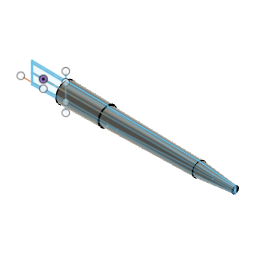
CustomDesignedTip_1000uL (Autodesk Fusion 360 design; units mm, degrees)
Autodesk Fusion 360 part; units mm, degrees
sketch "Sketch1" plane through (0, 0, 0) normal (0, 1, 0) x (1, 0, 0)
  line L0 (85.3, -0.9) -> (85.3, 0.9)
  line L1 (85.3, -1.4) -> (85.3, 1.4)
  line L2 (0, 0) -> (28.5, 0) construction
  line L3 (85.3, 0) -> (69.3, 0) construction
  line L4 (28.5, -4.086) -> (28.5, 4.086) construction
  line L5 (0, 0) -> (10, 0) construction
  line L6 (0, 3.75) -> (-10.0015, 3.75) construction
  line L7 (10, -3) -> (10, 3) construction
  line L8 (69.3, -3) -> (69.3, 3) construction
  line L9 (85.3, -0.9) -> (75.3, -0.9)
  line L10 (10, 3) -> (33, 3)
  line L11 (10, -3) -> (33, -3)
  line L12 (33, -3) -> (75.3, -0.9)
  line L13 (85.3, 0.9) -> (75.3, 0.9)
  line L14 (33, 3) -> (75.3, 0.9)
  line L15 (69.3, -3) -> (85.3, -1.4)
  line L16 (69.3, 3) -> (85.3, 1.4)
  line L17 (28.5, 4.086) -> (28.5, 3.736)
  line L18 (28.5, -4.086) -> (28.5, -3.736)
  line L19 (28.5, 3.736) -> (69.3, 3)
  line L20 (28.5, -3.736) -> (69.3, -3)
  line L21 (85.3, 0) -> (-5, 0)
  line L22 (-5, -4.6) -> (-5, 4.6)
  line L23 (-5, -3.75) -> (-5, 3.75)
  line L24 (-5, 0) -> (10, 0) construction
  line L25 (10, -8) -> (10, 8)
  line L26 (-5, -3.75) -> (10, -3.4882)
  line L27 (-5, -3.75) -> (10.0023, -3.75) construction
  line L28 (-5, 3.75) -> (10, 3.4882)
  line L29 (-5, 3.75) -> (10.0023, 3.75) construction
  line L30 (10, 3) -> (10, 3.4882)
  line L31 (10, -3.4882) -> (10, -3)
  line L32 (-5, -4.6) -> (28.5, -4.086)
  line L33 (-5, 4.6) -> (28.5, 4.086)
  line L34 (-5, 0) -> (28.5, 0) construction
  dimension "d4" = 1.8
  dimension "d5" = 2.8
  dimension "d7" = 16
  dimension "d9" = 8.172
  dimension "d15" = 6
  dimension "d16" = 6
  dimension "d17" = 10
  dimension "d18" = 23
  dimension "d21" = 0.35
  dimension "d22" = 0.35
  dimension "d25" = 90.3
  dimension "d26" = 9.2
  dimension "d27" = 7.5
  dimension "d28" = 15
  dimension "d29" = 1
  dimension "d31" = 33.5
  constraint vertical L0
  constraint midpoint L3.start L0
  constraint vertical L1
  constraint midpoint L3.start L1
  constraint coincident L2.start L5.start
  constraint perpendicular L0 L3
  constraint vertical L4
  constraint midpoint L2.end L4
  constraint horizontal L6
  constraint vertical L7
  constraint midpoint L5.end L7
  constraint vertical L8
  constraint midpoint L3.end L8
  constraint perpendicular L0 L9
  constraint equal L10 L11
  constraint perpendicular L0 L13
  constraint equal L9 L13
  constraint parallel L4 L17
  constraint coincident L4 L18.end
  constraint vertical L22
  constraint vertical L23
  constraint midpoint L21.end L22
  constraint midpoint L21.end L23
  constraint perpendicular L10 L25
  constraint midpoint L5.end L25
  constraint horizontal L27
  constraint coincident L25 L26.end
  constraint horizontal L29
  constraint coincident L25 L28.end
  constraint parallel L25 L30
  constraint perpendicular L11 L31
  constraint equal L26 L28
  constraint perpendicular L21 L23
  constraint perpendicular L4 L34
  measures "d4" distance of L0.start L0.end
  measures "d5" distance of L1.start L1.end
  measures "d7" distance of L3.start L3.end
  measures "d9" distance of L4.start L4.end
  measures "d15" distance of L7.start L7.end
  measures "d16" distance of L8.start L8.end
  measures "d17" distance of L0.start L9.end
  measures "d18" distance of L7.end L10.end
  measures "d21" distance of L4.end L17.end
  measures "d22" distance of L4.start L18.end
  measures "d25" distance of L3.start L21.end
  measures "d26" distance of L22.start L22.end
  measures "d27" distance of L23.start L23.end
  measures "d28" distance of L5.end L21.end
  measures "d29" angle of L26 L27
  measures "d31" distance of L2.end L21.end
revolve "Revolve4" add sketch "Sketch1" angle 360 about axis through (85.3, 0, 0) along (-1, 0, 0) contours L1 L10 L13 L14 L16 L17 L19 L25 L30 L33
